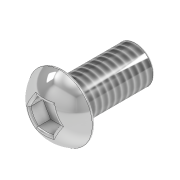
# Autodesk Inventor part: M4 x 8 Pin Head Allen Bolt
Saved by Autodesk Inventor 2020 (Build 240168000, 168)
## iProperties
Created: 2021-07-31
Part Number: M4 x 8 Pin Head Allen Bolt
Material: Generic
Document SubType Name: Modeling
Designer: Coy
Density: 1 g/cm^3
Appearance: Chrome - Polished
Author: Coy
Autodesk Inventor part; units mm, degrees
ref_plane "YZ Plane" through (0, 0, 0) normal (1, 0, 0) x (0, 1, 0)
ref_plane "XZ Plane" through (0, 0, 0) normal (0, 1, 0) x (-1, 0, 0)
ref_plane "XY Plane" through (0, 0, 0) normal (0, 0, 1) x (1, 0, 0)
sketch "Sketch1" plane through (0, 0, 0) normal (1, 0, 0) x (0, 1, 0)
  line L0 (0, 0) -> (2, 0)
  line L1 (2, 0) -> (2, 8)
  line L2 (2, 8) -> (3.6, 8)
  line L3 (8.1636, 10.5) -> (-8.3187, 10.5) construction
  line L4 (0, 0) -> (0, 10.5)
  arc A0 (3.6, 8) -> (0, 10.5) centre (0, 6.658) ccw
  dimension "d0" = 2
  dimension "d1" = 8
  dimension "d2" = 1.6
  dimension "d3" = 2.5
  constraints: 10 end point, 3 perpendicular, 2 horizontal, 2 point on circle, 1 centre point, 1 point on line, 1 tangent
  measures "d0" distance of L0.start L0.end
  measures "d1" distance of L0.end L1.end
  measures "d2" distance of L1.end L2.end
  measures "d3" distance between parallel lines of L2 L3
revolve "Revolution1" add sketch "Sketch1" angle 360 about axis through (0, 0, 0) along (0, 0, 1)
ref_plane "Work Plane1" through (0, 0, 10.5) normal (0, 0, -1) x (-1, 0, 0)
sketch "Sketch2" plane through (0, 0, 10.5) normal (0, 0, -1) x (-1, 0, 0)
  line L0 (0.8372, 1.45) -> (1.6743, 0)
  line L1 (1.6743, 0) -> (0.8372, -1.45)
  line L2 (0.8372, -1.45) -> (-0.8372, -1.45)
  line L3 (-0.8372, -1.45) -> (-1.6743, 0)
  line L4 (-1.6743, 0) -> (-0.8372, 1.45)
  line L5 (-0.8372, 1.45) -> (0.8372, 1.45)
  point P0 (0, 0)
  point P1 (0, 0)
  dimension "d6" = 1.45
  constraints: 12 end point, 1 coincident, 13 other
  measures "d6" distance from line of point (0, 0) L5
extrude "Extrusion1" cut sketch "Sketch2" along normal blind 2
fillet "Fillet1" radius 0.2 10 edges at (1.2557, -0.725, 10.2159) (0, -1.45, 10.2159) (-1.2557, -0.725, 10.2159) (-1.2557, 0.725, 10.2159) (-0.4215, 1.45, 10.1908) (0.4215, 1.45, 10.1908) (1.2557, 0.725, 10.2159) (0, -3.6, 8) (0, -2, 8) (0, -2, 0)
thread "Thread1" size "M4x0.7" class "6g" standard "ANSI Metric M Profile" full length
body "Solid1"
